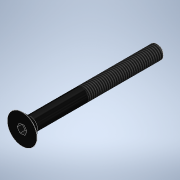
# Autodesk Inventor part: SCREW,FLAT HD,P, 5,M8X1.25X80MM
Saved by Autodesk Inventor 2022.4 (Build 264492000, 492)
## iProperties
Category: _
Manager: 100-64242
Created: 2001-02-21
Part Number: SCREW,FLAT HD,P, 5,M8X1.25X80MM
Material: Default
Document SubType Name: Modeling
Designer: cdotson
Description: SCREW,FLAT HD,P, 5,M8X1.25X80MM
Density: 1 g/cm^3
Appearance: Glossy - Black
Checked By: 0001253399
User Status: Work In Process
Engr Approved By: P
Mfg Approved By: -
Mass: 4.38503 g
Surface Area: 24.9953 cm^2
Volume: 4.38503 cm^3
Control State: 0
Master: False
Checked Out: False
Shininess: 64.0
Length Units: 11269
Angle Units: 11279
Time Units: 11290
Mass Units: 11283
Length Display Precision: 3
Angle Display Precision: 2
PTC_WM_ITERATION: 1
PTC_WM_ORGANIZATION_ID: CLWC
PTC_WM_LIFECYCLE: CLWC_CAD_LC
FIRST_DESCRIPTION: _
SECOND_DESCRIPTION: _
THIRD_DESCRIPTION: _
CN_MASS: 0.00438502880016333
CL_runCount: 1
FinishProperty: ToBeSet
CN_Serviceable: _
ModelCat: Uncategorized
Density: 0.0
Volumn: 0.0
Area: 0.0
PropertySet Name: Model Information
Author: -
Revision Number: A
Subject: _
Keywords: -
Autodesk Inventor part; units mm, degrees
ref_plane "YZ Plane" through (0, 0, 0) normal (1, 0, 0) x (0, 1, 0)
ref_plane "XZ Plane" through (0, 0, 0) normal (0, 1, 0) x (-1, 0, 0)
ref_plane "XY Plane" through (0, 0, 0) normal (0, 0, 1) x (1, 0, 0)
sketch "Sketch1" plane through (0, 0, 0) normal (0, 0, 1) x (1, 0, 0)
  circle A0 centre (0, 0) radius 4
  dimension "Diameter" = 8
  constraints: 1 centre point
  measures "Diameter" diameter of A0
extrude "Extrusion1" add sketch "Sketch1" along normal blind 75.04
sketch "Sketch2" plane through (0, 0, 75.04) normal (0, 0, 1) x (1, 0, 0)
  circle A0 centre (0, 0) radius 4 projected
extrude "Extrusion2" add sketch "Sketch2" along normal blind 4.96 draft 45
sketch "Sketch3" plane through (0, 0, 80) normal (0, 0, 1) x (1, 0, 0)
  circle A0 centre (0, 0) radius 8.96 projected
  circle A1 centre (0, 0) radius 2.8868 construction
  line L0 (1.2084, 2.6217) -> (2.8746, 0.2644)
  line L1 (2.8746, 0.2644) -> (1.6662, -2.3573)
  line L2 (1.6662, -2.3573) -> (-1.2084, -2.6217)
  line L3 (-1.2084, -2.6217) -> (-2.8746, -0.2644)
  line L4 (-2.8746, -0.2644) -> (-1.6662, 2.3573)
  line L5 (-1.6662, 2.3573) -> (1.2084, 2.6217)
  dimension "Hex_Width" = 5
  constraints: 12 end point, 6 point on circle, 4 equal length, 1 centre point, 1 coincident
  measures "Hex_Width" distance between parallel lines of L0 L3
extrude "Extrusion3" cut sketch "Sketch3" against normal blind 3 contours L0 L1 L2 L3 L4 L5
thread "Thread1" size "M8x1.25" class "4g6g" standard "ANSI Metric M Profile" length 45
chamfer "Chamfer2" distance 0.8 angle 45 1 edges at (-4, 0, 0)
fillet "Fillet1" radius 0.1 1 edges at (-8.96, 0, 80)
equation "\"d10\" = Thread_Length"
equation "\"d13\" = Chamfer"
equation "\"Thread_Length\" = 45"
equation "\"Chamfer\" = 0.8"
body "Solid1"
